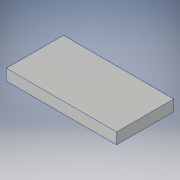
# Autodesk Inventor part: Gehaeuse_Deckel
Saved by Autodesk Inventor 2019 (Build 230136000, 136)
## iProperties
Created: 2019-01-15
Part Number: Gehaeuse_Deckel
Material: Generic
Document SubType Name: Modeling
Designer: patri
Density: 1 g/cm^3
Appearance: Aluminum - Flat
Author: patri
Autodesk Inventor part; units mm, degrees
ref_plane "YZ Plane" through (0, 0, 0) normal (1, 0, 0) x (0, 1, 0)
ref_plane "XZ Plane" through (0, 0, 0) normal (0, 1, 0) x (-1, 0, 0)
ref_plane "XY Plane" through (0, 0, 0) normal (0, 0, 1) x (1, 0, 0)
sketch "Sketch1" plane through (0, 0, 0) normal (0, 1, 0) x (-1, 0, 0)
  line L0 (222, -115) -> (-222, -115)
  line L1 (-222, -115) -> (-222, 115)
  line L2 (-222, 115) -> (222, 115)
  line L3 (222, 115) -> (222, -115)
  line L4 (0, -161) -> (0, 161) projected
  line L5 (310.8, 0) -> (-310.8, 0) projected
  point P0 (0, 0)
  dimension "d0" = 444
  dimension "d1" = 230
  constraints: 8 end point, 2 parallel, 1 horizontal, 1 perpendicular, 2 other
  measures "d0" distance of L0.start L0.end
  measures "d1" distance of L0.end L1.end
extrude "Extrusion1" add sketch "Sketch1" along normal blind 45
sketch "Sketch10" plane through (0, 0, 0) normal (0, -1, 0) x (1, 0, 0)
  line L0 (-221.88, 114.88) -> (221.88, 114.88)
  line L1 (221.88, 114.88) -> (221.88, -114.88)
  line L2 (221.88, -114.88) -> (-221.88, -114.88)
  line L3 (-221.88, -114.88) -> (-221.88, 114.88)
  line L4 (0, -161) -> (0, 161) projected
  line L5 (-310.8, 0) -> (310.8, 0) projected
  line L6 (-222, 115) -> (-222, -115) projected
  line L7 (222, 115) -> (-222, 115) projected
  point P0 (0, 0)
  dimension "d19" = 0.12
  dimension "d20" = 0.12
  constraints: 8 end point, 2 parallel, 1 horizontal, 1 perpendicular, 2 other
  measures "d19" distance between parallel lines of L3 L6
  measures "d20" distance between parallel lines of L0 L7
extrude "Extrusion6" cut sketch "Sketch10" against normal blind 44.88 contours L0 L4 L5 L3 | L0 L1 L5 L4 | L5 L4 L2 L3 | L5 L1 L2 L4
body "Solid1"
